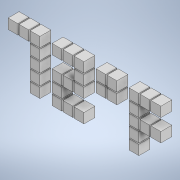
# Autodesk Inventor part: Sun Icon Mockup
Saved by Autodesk Inventor 2020 (Build 240168000, 168)
## iProperties
Created: 2021-04-14
Part Number: Sun Icon Mockup
Material: Generic
Document SubType Name: Modeling
Designer: user
Density: 1 g/cm^3
Appearance: Default
Author: user
Autodesk Inventor part; units mm, degrees
ref_plane "YZ Plane" through (0, 0, 0) normal (1, 0, 0) x (0, 1, 0)
ref_plane "XZ Plane" through (0, 0, 0) normal (0, 1, 0) x (-1, 0, 0)
ref_plane "XY Plane" through (0, 0, 0) normal (0, 0, 1) x (1, 0, 0)
sketch "Sketch1" plane through (0, 0, 0) normal (0, 0, 1) x (1, 0, 0)
  line L0 (0, 0) -> (9, 0)
  line L1 (9, 0) -> (9, 9)
  line L2 (9, 9) -> (0, 9)
  line L3 (0, 9) -> (0, 0)
  line L4 (10, 0) -> (19, 0)
  line L5 (19, 0) -> (19, 9)
  line L6 (10, 9) -> (10, 0)
  line L7 (19, 9) -> (10, 9)
  line L8 (20, 0) -> (29, 0)
  line L9 (29, 0) -> (29, 9)
  line L10 (20, 9) -> (20, 0)
  line L11 (29, 9) -> (20, 9)
  line L12 (30, 0) -> (39, 0)
  line L13 (39, 0) -> (39, 9)
  line L14 (30, 9) -> (30, 0)
  line L15 (39, 9) -> (30, 9)
  line L16 (40, 0) -> (49, 0)
  line L17 (49, 0) -> (49, 9)
  line L18 (40, 9) -> (40, 0)
  line L19 (49, 9) -> (40, 9)
  line L20 (50, 0) -> (59, 0)
  line L21 (59, 0) -> (59, 9)
  line L22 (50, 9) -> (50, 0)
  line L23 (59, 9) -> (50, 9)
  line L24 (60, 0) -> (69, 0)
  line L25 (69, 0) -> (69, 9)
  line L26 (60, 9) -> (60, 0)
  line L27 (69, 9) -> (60, 9)
  line L28 (70, 0) -> (79, 0)
  line L29 (79, 0) -> (79, 9)
  line L30 (70, 9) -> (70, 0)
  line L31 (79, 9) -> (70, 9)
  line L32 (80, 0) -> (89, 0)
  line L33 (89, 0) -> (89, 9)
  line L34 (80, 9) -> (80, 0)
  line L35 (89, 9) -> (80, 9)
  line L36 (90, 0) -> (99, 0)
  line L37 (99, 0) -> (99, 9)
  line L38 (90, 9) -> (90, 0)
  line L39 (99, 9) -> (90, 9)
  line L40 (100, 0) -> (109, 0)
  line L41 (109, 0) -> (109, 9)
  line L42 (100, 9) -> (100, 0)
  line L43 (109, 9) -> (100, 9)
  line L44 (110, 0) -> (119, 0)
  line L45 (119, 0) -> (119, 9)
  line L46 (110, 9) -> (110, 0)
  line L47 (119, 9) -> (110, 9)
  line L48 (120, 0) -> (129, 0)
  line L49 (129, 0) -> (129, 9)
  line L50 (120, 9) -> (120, 0)
  line L51 (129, 9) -> (120, 9)
  line L52 (130, 0) -> (139, 0)
  line L53 (139, 0) -> (139, 9)
  line L54 (130, 9) -> (130, 0)
  line L55 (139, 9) -> (130, 9)
  line L56 (140, 0) -> (149, 0)
  line L57 (149, 0) -> (149, 9)
  line L58 (140, 9) -> (140, 0)
  line L59 (149, 9) -> (140, 9)
  line L60 (150, 0) -> (159, 0)
  line L61 (159, 0) -> (159, 9)
  line L62 (150, 9) -> (150, 0)
  line L63 (159, 9) -> (150, 9)
  line L64 (160, 0) -> (169, 0)
  line L65 (169, 0) -> (169, 9)
  line L66 (160, 9) -> (160, 0)
  line L67 (169, 9) -> (160, 9)
  line L68 (170, 0) -> (179, 0)
  line L69 (179, 0) -> (179, 9)
  line L70 (170, 9) -> (170, 0)
  line L71 (179, 9) -> (170, 9)
  line L72 (180, 0) -> (189, 0)
  line L73 (189, 0) -> (189, 9)
  line L74 (180, 9) -> (180, 0)
  line L75 (189, 9) -> (180, 9)
  line L76 (190, 0) -> (199, 0)
  line L77 (199, 0) -> (199, 9)
  line L78 (190, 9) -> (190, 0)
  line L79 (199, 9) -> (190, 9)
  line L80 (200, 0) -> (209, 0)
  line L81 (209, 0) -> (209, 9)
  line L82 (200, 9) -> (200, 0)
  line L83 (209, 9) -> (200, 9)
  line L84 (210, 0) -> (219, 0)
  line L85 (219, 0) -> (219, 9)
  line L86 (210, 9) -> (210, 0)
  line L87 (219, 9) -> (210, 9)
  line L88 (220, 0) -> (229, 0)
  line L89 (229, 0) -> (229, 9)
  line L90 (220, 9) -> (220, 0)
  line L91 (229, 9) -> (220, 9)
  line L92 (230, 0) -> (239, 0)
  line L93 (239, 0) -> (239, 9)
  line L94 (230, 9) -> (230, 0)
  line L95 (239, 9) -> (230, 9)
  line L96 (240, 0) -> (249, 0)
  line L97 (249, 0) -> (249, 9)
  line L98 (240, 9) -> (240, 0)
  line L99 (249, 9) -> (240, 9)
  line L100 (250, 0) -> (259, 0)
  line L101 (259, 0) -> (259, 9)
  line L102 (250, 9) -> (250, 0)
  line L103 (259, 9) -> (250, 9)
  line L104 (260, 0) -> (269, 0)
  line L105 (269, 0) -> (269, 9)
  line L106 (260, 9) -> (260, 0)
  line L107 (269, 9) -> (260, 9)
  line L108 (270, 0) -> (279, 0)
  line L109 (279, 0) -> (279, 9)
  line L110 (270, 9) -> (270, 0)
  line L111 (279, 9) -> (270, 9)
  line L112 (280, 0) -> (289, 0)
  line L113 (289, 0) -> (289, 9)
  line L114 (280, 9) -> (280, 0)
  line L115 (289, 9) -> (280, 9)
  line L116 (290, 0) -> (299, 0)
  line L117 (299, 0) -> (299, 9)
  line L118 (290, 9) -> (290, 0)
  line L119 (299, 9) -> (290, 9)
  line L120 (300, 0) -> (309, 0)
  line L121 (309, 0) -> (309, 9)
  line L122 (300, 9) -> (300, 0)
  line L123 (309, 9) -> (300, 9)
  line L124 (310, 0) -> (319, 0)
  line L125 (319, 0) -> (319, 9)
  line L126 (310, 9) -> (310, 0)
  line L127 (319, 9) -> (310, 9)
  line L128 (0, -10) -> (9, -10)
  line L129 (9, -10) -> (9, -1)
  line L130 (0, -1) -> (0, -10)
  line L131 (9, -1) -> (0, -1)
  line L132 (10, -10) -> (19, -10)
  line L133 (19, -10) -> (19, -1)
  line L134 (10, -1) -> (10, -10)
  line L135 (19, -1) -> (10, -1)
  line L136 (20, -10) -> (29, -10)
  line L137 (29, -10) -> (29, -1)
  line L138 (20, -1) -> (20, -10)
  line L139 (29, -1) -> (20, -1)
  line L140 (30, -10) -> (39, -10)
  line L141 (39, -10) -> (39, -1)
  line L142 (30, -1) -> (30, -10)
  line L143 (39, -1) -> (30, -1)
  line L144 (40, -10) -> (49, -10)
  line L145 (49, -10) -> (49, -1)
  line L146 (40, -1) -> (40, -10)
  line L147 (49, -1) -> (40, -1)
  line L148 (50, -10) -> (59, -10)
  line L149 (59, -10) -> (59, -1)
  line L150 (50, -1) -> (50, -10)
  line L151 (59, -1) -> (50, -1)
  line L152 (60, -10) -> (69, -10)
  line L153 (69, -10) -> (69, -1)
  line L154 (60, -1) -> (60, -10)
  line L155 (69, -1) -> (60, -1)
  line L156 (70, -10) -> (79, -10)
  line L157 (79, -10) -> (79, -1)
  line L158 (70, -1) -> (70, -10)
  line L159 (79, -1) -> (70, -1)
  line L160 (80, -10) -> (89, -10)
  line L161 (89, -10) -> (89, -1)
  line L162 (80, -1) -> (80, -10)
  line L163 (89, -1) -> (80, -1)
  line L164 (90, -10) -> (99, -10)
  line L165 (99, -10) -> (99, -1)
  line L166 (90, -1) -> (90, -10)
  line L167 (99, -1) -> (90, -1)
  line L168 (100, -10) -> (109, -10)
  line L169 (109, -10) -> (109, -1)
  line L170 (100, -1) -> (100, -10)
  line L171 (109, -1) -> (100, -1)
  line L172 (110, -10) -> (119, -10)
  line L173 (119, -10) -> (119, -1)
  line L174 (110, -1) -> (110, -10)
  line L175 (119, -1) -> (110, -1)
  line L176 (120, -10) -> (129, -10)
  line L177 (129, -10) -> (129, -1)
  line L178 (120, -1) -> (120, -10)
  line L179 (129, -1) -> (120, -1)
  line L180 (130, -10) -> (139, -10)
  line L181 (139, -10) -> (139, -1)
  line L182 (130, -1) -> (130, -10)
  line L183 (139, -1) -> (130, -1)
  line L184 (140, -10) -> (149, -10)
  line L185 (149, -10) -> (149, -1)
  line L186 (140, -1) -> (140, -10)
  line L187 (149, -1) -> (140, -1)
  line L188 (150, -10) -> (159, -10)
  line L189 (159, -10) -> (159, -1)
  line L190 (150, -1) -> (150, -10)
  line L191 (159, -1) -> (150, -1)
  line L192 (160, -10) -> (169, -10)
  line L193 (169, -10) -> (169, -1)
  line L194 (160, -1) -> (160, -10)
  line L195 (169, -1) -> (160, -1)
  line L196 (170, -10) -> (179, -10)
  line L197 (179, -10) -> (179, -1)
  line L198 (170, -1) -> (170, -10)
  line L199 (179, -1) -> (170, -1)
  line L200 (180, -10) -> (189, -10)
  line L201 (189, -10) -> (189, -1)
  line L202 (180, -1) -> (180, -10)
  line L203 (189, -1) -> (180, -1)
  line L204 (190, -10) -> (199, -10)
  line L205 (199, -10) -> (199, -1)
  line L206 (190, -1) -> (190, -10)
  line L207 (199, -1) -> (190, -1)
  line L208 (200, -10) -> (209, -10)
  line L209 (209, -10) -> (209, -1)
  line L210 (200, -1) -> (200, -10)
  line L211 (209, -1) -> (200, -1)
  line L212 (210, -10) -> (219, -10)
  line L213 (219, -10) -> (219, -1)
  line L214 (210, -1) -> (210, -10)
  line L215 (219, -1) -> (210, -1)
  line L216 (220, -10) -> (229, -10)
  line L217 (229, -10) -> (229, -1)
  line L218 (220, -1) -> (220, -10)
  line L219 (229, -1) -> (220, -1)
  line L220 (230, -10) -> (239, -10)
  line L221 (239, -10) -> (239, -1)
  line L222 (230, -1) -> (230, -10)
  line L223 (239, -1) -> (230, -1)
  line L224 (240, -10) -> (249, -10)
  line L225 (249, -10) -> (249, -1)
  line L226 (240, -1) -> (240, -10)
  line L227 (249, -1) -> (240, -1)
  line L228 (250, -10) -> (259, -10)
  line L229 (259, -10) -> (259, -1)
  line L230 (250, -1) -> (250, -10)
  line L231 (259, -1) -> (250, -1)
  line L232 (260, -10) -> (269, -10)
  line L233 (269, -10) -> (269, -1)
  line L234 (260, -1) -> (260, -10)
  line L235 (269, -1) -> (260, -1)
  line L236 (270, -10) -> (279, -10)
  line L237 (279, -10) -> (279, -1)
  line L238 (270, -1) -> (270, -10)
  line L239 (279, -1) -> (270, -1)
  line L240 (280, -10) -> (289, -10)
  line L241 (289, -10) -> (289, -1)
  line L242 (280, -1) -> (280, -10)
  line L243 (289, -1) -> (280, -1)
  line L244 (290, -10) -> (299, -10)
  line L245 (299, -10) -> (299, -1)
  line L246 (290, -1) -> (290, -10)
  line L247 (299, -1) -> (290, -1)
  line L248 (300, -10) -> (309, -10)
  line L249 (309, -10) -> (309, -1)
  line L250 (300, -1) -> (300, -10)
  line L251 (309, -1) -> (300, -1)
  line L252 (310, -10) -> (319, -10)
  line L253 (319, -10) -> (319, -1)
  line L254 (310, -1) -> (310, -10)
  line L255 (319, -1) -> (310, -1)
  line L256 (0, -20) -> (9, -20)
  line L257 (9, -20) -> (9, -11)
  line L258 (0, -11) -> (0, -20)
  line L259 (9, -11) -> (0, -11)
  line L260 (10, -20) -> (19, -20)
  line L261 (19, -20) -> (19, -11)
  line L262 (10, -11) -> (10, -20)
  line L263 (19, -11) -> (10, -11)
  line L264 (20, -20) -> (29, -20)
  line L265 (29, -20) -> (29, -11)
  line L266 (20, -11) -> (20, -20)
  line L267 (29, -11) -> (20, -11)
  line L268 (30, -20) -> (39, -20)
  line L269 (39, -20) -> (39, -11)
  line L270 (30, -11) -> (30, -20)
  line L271 (39, -11) -> (30, -11)
  line L272 (40, -20) -> (49, -20)
  line L273 (49, -20) -> (49, -11)
  line L274 (40, -11) -> (40, -20)
  line L275 (49, -11) -> (40, -11)
  line L276 (50, -20) -> (59, -20)
  line L277 (59, -20) -> (59, -11)
  line L278 (50, -11) -> (50, -20)
  line L279 (59, -11) -> (50, -11)
  line L280 (60, -20) -> (69, -20)
  line L281 (69, -20) -> (69, -11)
  line L282 (60, -11) -> (60, -20)
  line L283 (69, -11) -> (60, -11)
  line L284 (70, -20) -> (79, -20)
  line L285 (79, -20) -> (79, -11)
  line L286 (70, -11) -> (70, -20)
  line L287 (79, -11) -> (70, -11)
  line L288 (80, -20) -> (89, -20)
  line L289 (89, -20) -> (89, -11)
  line L290 (80, -11) -> (80, -20)
  line L291 (89, -11) -> (80, -11)
  line L292 (90, -20) -> (99, -20)
  line L293 (99, -20) -> (99, -11)
  line L294 (90, -11) -> (90, -20)
  line L295 (99, -11) -> (90, -11)
  line L296 (100, -20) -> (109, -20)
  line L297 (109, -20) -> (109, -11)
  line L298 (100, -11) -> (100, -20)
  line L299 (109, -11) -> (100, -11)
  line L300 (110, -20) -> (119, -20)
  line L301 (119, -20) -> (119, -11)
  line L302 (110, -11) -> (110, -20)
  line L303 (119, -11) -> (110, -11)
  line L304 (120, -20) -> (129, -20)
  line L305 (129, -20) -> (129, -11)
  line L306 (120, -11) -> (120, -20)
  line L307 (129, -11) -> (120, -11)
  line L308 (130, -20) -> (139, -20)
  line L309 (139, -20) -> (139, -11)
  line L310 (130, -11) -> (130, -20)
  line L311 (139, -11) -> (130, -11)
  line L312 (140, -20) -> (149, -20)
  line L313 (149, -20) -> (149, -11)
  line L314 (140, -11) -> (140, -20)
  line L315 (149, -11) -> (140, -11)
  line L316 (150, -20) -> (159, -20)
  line L317 (159, -20) -> (159, -11)
  line L318 (150, -11) -> (150, -20)
  line L319 (159, -11) -> (150, -11)
  line L320 (160, -20) -> (169, -20)
  line L321 (169, -20) -> (169, -11)
  line L322 (160, -11) -> (160, -20)
  line L323 (169, -11) -> (160, -11)
  line L324 (170, -20) -> (179, -20)
  line L325 (179, -20) -> (179, -11)
  line L326 (170, -11) -> (170, -20)
  line L327 (179, -11) -> (170, -11)
  line L328 (180, -20) -> (189, -20)
  line L329 (189, -20) -> (189, -11)
  line L330 (180, -11) -> (180, -20)
  line L331 (189, -11) -> (180, -11)
  line L332 (190, -20) -> (199, -20)
  line L333 (199, -20) -> (199, -11)
  line L334 (190, -11) -> (190, -20)
  line L335 (199, -11) -> (190, -11)
  line L336 (200, -20) -> (209, -20)
  line L337 (209, -20) -> (209, -11)
  line L338 (200, -11) -> (200, -20)
  line L339 (209, -11) -> (200, -11)
  line L340 (210, -20) -> (219, -20)
  line L341 (219, -20) -> (219, -11)
  line L342 (210, -11) -> (210, -20)
  line L343 (219, -11) -> (210, -11)
  line L344 (220, -20) -> (229, -20)
  line L345 (229, -20) -> (229, -11)
  line L346 (220, -11) -> (220, -20)
  line L347 (229, -11) -> (220, -11)
  line L348 (230, -20) -> (239, -20)
  line L349 (239, -20) -> (239, -11)
  line L350 (230, -11) -> (230, -20)
  line L351 (239, -11) -> (230, -11)
  line L352 (240, -20) -> (249, -20)
  line L353 (249, -20) -> (249, -11)
  line L354 (240, -11) -> (240, -20)
  line L355 (249, -11) -> (240, -11)
  line L356 (250, -20) -> (259, -20)
  line L357 (259, -20) -> (259, -11)
  line L358 (250, -11) -> (250, -20)
  line L359 (259, -11) -> (250, -11)
  line L360 (260, -20) -> (269, -20)
  line L361 (269, -20) -> (269, -11)
  line L362 (260, -11) -> (260, -20)
  line L363 (269, -11) -> (260, -11)
  line L364 (270, -20) -> (279, -20)
  line L365 (279, -20) -> (279, -11)
  line L366 (270, -11) -> (270, -20)
  line L367 (279, -11) -> (270, -11)
  line L368 (280, -20) -> (289, -20)
  line L369 (289, -20) -> (289, -11)
  line L370 (280, -11) -> (280, -20)
  line L371 (289, -11) -> (280, -11)
  line L372 (290, -20) -> (299, -20)
  line L373 (299, -20) -> (299, -11)
  line L374 (290, -11) -> (290, -20)
  line L375 (299, -11) -> (290, -11)
  line L376 (300, -20) -> (309, -20)
  line L377 (309, -20) -> (309, -11)
  line L378 (300, -11) -> (300, -20)
  line L379 (309, -11) -> (300, -11)
  line L380 (310, -20) -> (319, -20)
  line L381 (319, -20) -> (319, -11)
  line L382 (310, -11) -> (310, -20)
  line L383 (319, -11) -> (310, -11)
  line L384 (0, -30) -> (9, -30)
  line L385 (9, -30) -> (9, -21)
  line L386 (0, -21) -> (0, -30)
  line L387 (9, -21) -> (0, -21)
  line L388 (10, -30) -> (19, -30)
  line L389 (19, -30) -> (19, -21)
  line L390 (10, -21) -> (10, -30)
  line L391 (19, -21) -> (10, -21)
  line L392 (20, -30) -> (29, -30)
  line L393 (29, -30) -> (29, -21)
  line L394 (20, -21) -> (20, -30)
  line L395 (29, -21) -> (20, -21)
  line L396 (30, -30) -> (39, -30)
  line L397 (39, -30) -> (39, -21)
  line L398 (30, -21) -> (30, -30)
  line L399 (39, -21) -> (30, -21)
  line L400 (40, -30) -> (49, -30)
  line L401 (49, -30) -> (49, -21)
  line L402 (40, -21) -> (40, -30)
  line L403 (49, -21) -> (40, -21)
  line L404 (50, -30) -> (59, -30)
  line L405 (59, -30) -> (59, -21)
  line L406 (50, -21) -> (50, -30)
  line L407 (59, -21) -> (50, -21)
  line L408 (60, -30) -> (69, -30)
  line L409 (69, -30) -> (69, -21)
  line L410 (60, -21) -> (60, -30)
  line L411 (69, -21) -> (60, -21)
  line L412 (70, -30) -> (79, -30)
  line L413 (79, -30) -> (79, -21)
  line L414 (70, -21) -> (70, -30)
  line L415 (79, -21) -> (70, -21)
  line L416 (80, -30) -> (89, -30)
  line L417 (89, -30) -> (89, -21)
  line L418 (80, -21) -> (80, -30)
  line L419 (89, -21) -> (80, -21)
  line L420 (90, -30) -> (99, -30)
  line L421 (99, -30) -> (99, -21)
  line L422 (90, -21) -> (90, -30)
  line L423 (99, -21) -> (90, -21)
  line L424 (100, -30) -> (109, -30)
  line L425 (109, -30) -> (109, -21)
  line L426 (100, -21) -> (100, -30)
  line L427 (109, -21) -> (100, -21)
  line L428 (110, -30) -> (119, -30)
  line L429 (119, -30) -> (119, -21)
  line L430 (110, -21) -> (110, -30)
  line L431 (119, -21) -> (110, -21)
  line L432 (120, -30) -> (129, -30)
  line L433 (129, -30) -> (129, -21)
  line L434 (120, -21) -> (120, -30)
  line L435 (129, -21) -> (120, -21)
  line L436 (130, -30) -> (139, -30)
  line L437 (139, -30) -> (139, -21)
  line L438 (130, -21) -> (130, -30)
  line L439 (139, -21) -> (130, -21)
  line L440 (140, -30) -> (149, -30)
  line L441 (149, -30) -> (149, -21)
  line L442 (140, -21) -> (140, -30)
  line L443 (149, -21) -> (140, -21)
  line L444 (150, -30) -> (159, -30)
  line L445 (159, -30) -> (159, -21)
  line L446 (150, -21) -> (150, -30)
  line L447 (159, -21) -> (150, -21)
  line L448 (160, -30) -> (169, -30)
  line L449 (169, -30) -> (169, -21)
  line L450 (160, -21) -> (160, -30)
  line L451 (169, -21) -> (160, -21)
  line L452 (170, -30) -> (179, -30)
  line L453 (179, -30) -> (179, -21)
  line L454 (170, -21) -> (170, -30)
  line L455 (179, -21) -> (170, -21)
  line L456 (180, -30) -> (189, -30)
  line L457 (189, -30) -> (189, -21)
  line L458 (180, -21) -> (180, -30)
  line L459 (189, -21) -> (180, -21)
  line L460 (190, -30) -> (199, -30)
  line L461 (199, -30) -> (199, -21)
  line L462 (190, -21) -> (190, -30)
  line L463 (199, -21) -> (190, -21)
  line L464 (200, -30) -> (209, -30)
  line L465 (209, -30) -> (209, -21)
  line L466 (200, -21) -> (200, -30)
  line L467 (209, -21) -> (200, -21)
  line L468 (210, -30) -> (219, -30)
  line L469 (219, -30) -> (219, -21)
  line L470 (210, -21) -> (210, -30)
  line L471 (219, -21) -> (210, -21)
  line L472 (220, -30) -> (229, -30)
  line L473 (229, -30) -> (229, -21)
  line L474 (220, -21) -> (220, -30)
  line L475 (229, -21) -> (220, -21)
  line L476 (230, -30) -> (239, -30)
  line L477 (239, -30) -> (239, -21)
  line L478 (230, -21) -> (230, -30)
  line L479 (239, -21) -> (230, -21)
  line L480 (240, -30) -> (249, -30)
  line L481 (249, -30) -> (249, -21)
  line L482 (240, -21) -> (240, -30)
  line L483 (249, -21) -> (240, -21)
  line L484 (250, -30) -> (259, -30)
  line L485 (259, -30) -> (259, -21)
  line L486 (250, -21) -> (250, -30)
  line L487 (259, -21) -> (250, -21)
  line L488 (260, -30) -> (269, -30)
  line L489 (269, -30) -> (269, -21)
  line L490 (260, -21) -> (260, -30)
  line L491 (269, -21) -> (260, -21)
  line L492 (270, -30) -> (279, -30)
  line L493 (279, -30) -> (279, -21)
  line L494 (270, -21) -> (270, -30)
  line L495 (279, -21) -> (270, -21)
  line L496 (280, -30) -> (289, -30)
  line L497 (289, -30) -> (289, -21)
  line L498 (280, -21) -> (280, -30)
  line L499 (289, -21) -> (280, -21)
  line L500 (290, -30) -> (299, -30)
  line L501 (299, -30) -> (299, -21)
  line L502 (290, -21) -> (290, -30)
  line L503 (299, -21) -> (290, -21)
  line L504 (300, -30) -> (309, -30)
  line L505 (309, -30) -> (309, -21)
  line L506 (300, -21) -> (300, -30)
  line L507 (309, -21) -> (300, -21)
  line L508 (310, -30) -> (319, -30)
  line L509 (319, -30) -> (319, -21)
  line L510 (310, -21) -> (310, -30)
  line L511 (319, -21) -> (310, -21)
  line L512 (0, -40) -> (9, -40)
  line L513 (9, -40) -> (9, -31)
  line L514 (0, -31) -> (0, -40)
  line L515 (9, -31) -> (0, -31)
  line L516 (10, -40) -> (19, -40)
  line L517 (19, -40) -> (19, -31)
  line L518 (10, -31) -> (10, -40)
  line L519 (19, -31) -> (10, -31)
  line L520 (20, -40) -> (29, -40)
  line L521 (29, -40) -> (29, -31)
  line L522 (20, -31) -> (20, -40)
  line L523 (29, -31) -> (20, -31)
  line L524 (30, -40) -> (39, -40)
  line L525 (39, -40) -> (39, -31)
  line L526 (30, -31) -> (30, -40)
  line L527 (39, -31) -> (30, -31)
  line L528 (40, -40) -> (49, -40)
  line L529 (49, -40) -> (49, -31)
  line L530 (40, -31) -> (40, -40)
  line L531 (49, -31) -> (40, -31)
  line L532 (50, -40) -> (59, -40)
  line L533 (59, -40) -> (59, -31)
  line L534 (50, -31) -> (50, -40)
  line L535 (59, -31) -> (50, -31)
  line L536 (60, -40) -> (69, -40)
  line L537 (69, -40) -> (69, -31)
  line L538 (60, -31) -> (60, -40)
  line L539 (69, -31) -> (60, -31)
  line L540 (70, -40) -> (79, -40)
  line L541 (79, -40) -> (79, -31)
  line L542 (70, -31) -> (70, -40)
  line L543 (79, -31) -> (70, -31)
  line L544 (80, -40) -> (89, -40)
  line L545 (89, -40) -> (89, -31)
  line L546 (80, -31) -> (80, -40)
  line L547 (89, -31) -> (80, -31)
  line L548 (90, -40) -> (99, -40)
  line L549 (99, -40) -> (99, -31)
  line L550 (90, -31) -> (90, -40)
  line L551 (99, -31) -> (90, -31)
  line L552 (100, -40) -> (109, -40)
  line L553 (109, -40) -> (109, -31)
  line L554 (100, -31) -> (100, -40)
  line L555 (109, -31) -> (100, -31)
  line L556 (110, -40) -> (119, -40)
  line L557 (119, -40) -> (119, -31)
  line L558 (110, -31) -> (110, -40)
  line L559 (119, -31) -> (110, -31)
  line L560 (120, -40) -> (129, -40)
  line L561 (129, -40) -> (129, -31)
  line L562 (120, -31) -> (120, -40)
  line L563 (129, -31) -> (120, -31)
  line L564 (130, -40) -> (139, -40)
  line L565 (139, -40) -> (139, -31)
  line L566 (130, -31) -> (130, -40)
  line L567 (139, -31) -> (130, -31)
  line L568 (140, -40) -> (149, -40)
  line L569 (149, -40) -> (149, -31)
  line L570 (140, -31) -> (140, -40)
  line L571 (149, -31) -> (140, -31)
  line L572 (150, -40) -> (159, -40)
  line L573 (159, -40) -> (159, -31)
  line L574 (150, -31) -> (150, -40)
  line L575 (159, -31) -> (150, -31)
  line L576 (160, -40) -> (169, -40)
  line L577 (169, -40) -> (169, -31)
  line L578 (160, -31) -> (160, -40)
  line L579 (169, -31) -> (160, -31)
  line L580 (170, -40) -> (179, -40)
  line L581 (179, -40) -> (179, -31)
  line L582 (170, -31) -> (170, -40)
  line L583 (179, -31) -> (170, -31)
  line L584 (180, -40) -> (189, -40)
  line L585 (189, -40) -> (189, -31)
  line L586 (180, -31) -> (180, -40)
  line L587 (189, -31) -> (180, -31)
  line L588 (190, -40) -> (199, -40)
  line L589 (199, -40) -> (199, -31)
  line L590 (190, -31) -> (190, -40)
  line L591 (199, -31) -> (190, -31)
  line L592 (200, -40) -> (209, -40)
  line L593 (209, -40) -> (209, -31)
  line L594 (200, -31) -> (200, -40)
  line L595 (209, -31) -> (200, -31)
  line L596 (210, -40) -> (219, -40)
  line L597 (219, -40) -> (219, -31)
  line L598 (210, -31) -> (210, -40)
  line L599 (219, -31) -> (210, -31)
  line L600 (220, -40) -> (229, -40)
  line L601 (229, -40) -> (229, -31)
  line L602 (220, -31) -> (220, -40)
  line L603 (229, -31) -> (220, -31)
  line L604 (230, -40) -> (239, -40)
  line L605 (239, -40) -> (239, -31)
  line L606 (230, -31) -> (230, -40)
  line L607 (239, -31) -> (230, -31)
  line L608 (240, -40) -> (249, -40)
  line L609 (249, -40) -> (249, -31)
  line L610 (240, -31) -> (240, -40)
  line L611 (249, -31) -> (240, -31)
  line L612 (250, -40) -> (259, -40)
  line L613 (259, -40) -> (259, -31)
  line L614 (250, -31) -> (250, -40)
  line L615 (259, -31) -> (250, -31)
  line L616 (260, -40) -> (269, -40)
  line L617 (269, -40) -> (269, -31)
  line L618 (260, -31) -> (260, -40)
  line L619 (269, -31) -> (260, -31)
  line L620 (270, -40) -> (279, -40)
  line L621 (279, -40) -> (279, -31)
  line L622 (270, -31) -> (270, -40)
  line L623 (279, -31) -> (270, -31)
  line L624 (280, -40) -> (289, -40)
  line L625 (289, -40) -> (289, -31)
  line L626 (280, -31) -> (280, -40)
  line L627 (289, -31) -> (280, -31)
  line L628 (290, -40) -> (299, -40)
  line L629 (299, -40) -> (299, -31)
  line L630 (290, -31) -> (290, -40)
  line L631 (299, -31) -> (290, -31)
  line L632 (300, -40) -> (309, -40)
  line L633 (309, -40) -> (309, -31)
  line L634 (300, -31) -> (300, -40)
  line L635 (309, -31) -> (300, -31)
  line L636 (310, -40) -> (319, -40)
  line L637 (319, -40) -> (319, -31)
  line L638 (310, -31) -> (310, -40)
  line L639 (319, -31) -> (310, -31)
  line L640 (0, -50) -> (9, -50)
  line L641 (9, -50) -> (9, -41)
  line L642 (0, -41) -> (0, -50)
  line L643 (9, -41) -> (0, -41)
  line L644 (10, -50) -> (19, -50)
  line L645 (19, -50) -> (19, -41)
  line L646 (10, -41) -> (10, -50)
  line L647 (19, -41) -> (10, -41)
  line L648 (20, -50) -> (29, -50)
  line L649 (29, -50) -> (29, -41)
  line L650 (20, -41) -> (20, -50)
  line L651 (29, -41) -> (20, -41)
  line L652 (30, -50) -> (39, -50)
  line L653 (39, -50) -> (39, -41)
  line L654 (30, -41) -> (30, -50)
  line L655 (39, -41) -> (30, -41)
  line L656 (40, -50) -> (49, -50)
  line L657 (49, -50) -> (49, -41)
  line L658 (40, -41) -> (40, -50)
  line L659 (49, -41) -> (40, -41)
  line L660 (50, -50) -> (59, -50)
  line L661 (59, -50) -> (59, -41)
  line L662 (50, -41) -> (50, -50)
  line L663 (59, -41) -> (50, -41)
  line L664 (60, -50) -> (69, -50)
  line L665 (69, -50) -> (69, -41)
  line L666 (60, -41) -> (60, -50)
  line L667 (69, -41) -> (60, -41)
  line L668 (70, -50) -> (79, -50)
  line L669 (79, -50) -> (79, -41)
  line L670 (70, -41) -> (70, -50)
  line L671 (79, -41) -> (70, -41)
  line L672 (80, -50) -> (89, -50)
  line L673 (89, -50) -> (89, -41)
  line L674 (80, -41) -> (80, -50)
  line L675 (89, -41) -> (80, -41)
  line L676 (90, -50) -> (99, -50)
  line L677 (99, -50) -> (99, -41)
  line L678 (90, -41) -> (90, -50)
  line L679 (99, -41) -> (90, -41)
  line L680 (100, -50) -> (109, -50)
  line L681 (109, -50) -> (109, -41)
  line L682 (100, -41) -> (100, -50)
  line L683 (109, -41) -> (100, -41)
  line L684 (110, -50) -> (119, -50)
  line L685 (119, -50) -> (119, -41)
  line L686 (110, -41) -> (110, -50)
  line L687 (119, -41) -> (110, -41)
  line L688 (120, -50) -> (129, -50)
  line L689 (129, -50) -> (129, -41)
  line L690 (120, -41) -> (120, -50)
  line L691 (129, -41) -> (120, -41)
  line L692 (130, -50) -> (139, -50)
  line L693 (139, -50) -> (139, -41)
  line L694 (130, -41) -> (130, -50)
  line L695 (139, -41) -> (130, -41)
  line L696 (140, -50) -> (149, -50)
  line L697 (149, -50) -> (149, -41)
  line L698 (140, -41) -> (140, -50)
  line L699 (149, -41) -> (140, -41)
  line L700 (150, -50) -> (159, -50)
  line L701 (159, -50) -> (159, -41)
  line L702 (150, -41) -> (150, -50)
  line L703 (159, -41) -> (150, -41)
  line L704 (160, -50) -> (169, -50)
  line L705 (169, -50) -> (169, -41)
  line L706 (160, -41) -> (160, -50)
  line L707 (169, -41) -> (160, -41)
  line L708 (170, -50) -> (179, -50)
  line L709 (179, -50) -> (179, -41)
  line L710 (170, -41) -> (170, -50)
  line L711 (179, -41) -> (170, -41)
  line L712 (180, -50) -> (189, -50)
  line L713 (189, -50) -> (189, -41)
  line L714 (180, -41) -> (180, -50)
  line L715 (189, -41) -> (180, -41)
  line L716 (190, -50) -> (199, -50)
  line L717 (199, -50) -> (199, -41)
  line L718 (190, -41) -> (190, -50)
  line L719 (199, -41) -> (190, -41)
  line L720 (200, -50) -> (209, -50)
  line L721 (209, -50) -> (209, -41)
  line L722 (200, -41) -> (200, -50)
  line L723 (209, -41) -> (200, -41)
  line L724 (210, -50) -> (219, -50)
  line L725 (219, -50) -> (219, -41)
  line L726 (210, -41) -> (210, -50)
  line L727 (219, -41) -> (210, -41)
  line L728 (220, -50) -> (229, -50)
  line L729 (229, -50) -> (229, -41)
  line L730 (220, -41) -> (220, -50)
  line L731 (229, -41) -> (220, -41)
  line L732 (230, -50) -> (239, -50)
  line L733 (239, -50) -> (239, -41)
  line L734 (230, -41) -> (230, -50)
  line L735 (239, -41) -> (230, -41)
  line L736 (240, -50) -> (249, -50)
  line L737 (249, -50) -> (249, -41)
  line L738 (240, -41) -> (240, -50)
  line L739 (249, -41) -> (240, -41)
  line L740 (250, -50) -> (259, -50)
  line L741 (259, -50) -> (259, -41)
  line L742 (250, -41) -> (250, -50)
  line L743 (259, -41) -> (250, -41)
  line L744 (260, -50) -> (269, -50)
  line L745 (269, -50) -> (269, -41)
  line L746 (260, -41) -> (260, -50)
  line L747 (269, -41) -> (260, -41)
  line L748 (270, -50) -> (279, -50)
  line L749 (279, -50) -> (279, -41)
  line L750 (270, -41) -> (270, -50)
  line L751 (279, -41) -> (270, -41)
  line L752 (280, -50) -> (289, -50)
  line L753 (289, -50) -> (289, -41)
  line L754 (280, -41) -> (280, -50)
  line L755 (289, -41) -> (280, -41)
  line L756 (290, -50) -> (299, -50)
  line L757 (299, -50) -> (299, -41)
  line L758 (290, -41) -> (290, -50)
  line L759 (299, -41) -> (290, -41)
  line L760 (300, -50) -> (309, -50)
  line L761 (309, -50) -> (309, -41)
  line L762 (300, -41) -> (300, -50)
  line L763 (309, -41) -> (300, -41)
  line L764 (310, -50) -> (319, -50)
  line L765 (319, -50) -> (319, -41)
  line L766 (310, -41) -> (310, -50)
  line L767 (319, -41) -> (310, -41)
  line L768 (0, -60) -> (9, -60)
  line L769 (9, -60) -> (9, -51)
  line L770 (0, -51) -> (0, -60)
  line L771 (9, -51) -> (0, -51)
  line L772 (10, -60) -> (19, -60)
  line L773 (19, -60) -> (19, -51)
  line L774 (10, -51) -> (10, -60)
  line L775 (19, -51) -> (10, -51)
  line L776 (20, -60) -> (29, -60)
  line L777 (29, -60) -> (29, -51)
  line L778 (20, -51) -> (20, -60)
  line L779 (29, -51) -> (20, -51)
  line L780 (30, -60) -> (39, -60)
  line L781 (39, -60) -> (39, -51)
  line L782 (30, -51) -> (30, -60)
  line L783 (39, -51) -> (30, -51)
  line L784 (40, -60) -> (49, -60)
  line L785 (49, -60) -> (49, -51)
  line L786 (40, -51) -> (40, -60)
  line L787 (49, -51) -> (40, -51)
  line L788 (50, -60) -> (59, -60)
  line L789 (59, -60) -> (59, -51)
  line L790 (50, -51) -> (50, -60)
  line L791 (59, -51) -> (50, -51)
  line L792 (60, -60) -> (69, -60)
  line L793 (69, -60) -> (69, -51)
  line L794 (60, -51) -> (60, -60)
  line L795 (69, -51) -> (60, -51)
  line L796 (70, -60) -> (79, -60)
  line L797 (79, -60) -> (79, -51)
  line L798 (70, -51) -> (70, -60)
  line L799 (79, -51) -> (70, -51)
  line L800 (80, -60) -> (89, -60)
  line L801 (89, -60) -> (89, -51)
  line L802 (80, -51) -> (80, -60)
  line L803 (89, -51) -> (80, -51)
  line L804 (90, -60) -> (99, -60)
  line L805 (99, -60) -> (99, -51)
  line L806 (90, -51) -> (90, -60)
  line L807 (99, -51) -> (90, -51)
  line L808 (100, -60) -> (109, -60)
  line L809 (109, -60) -> (109, -51)
  line L810 (100, -51) -> (100, -60)
  line L811 (109, -51) -> (100, -51)
  line L812 (110, -60) -> (119, -60)
  line L813 (119, -60) -> (119, -51)
  line L814 (110, -51) -> (110, -60)
  line L815 (119, -51) -> (110, -51)
  line L816 (120, -60) -> (129, -60)
  line L817 (129, -60) -> (129, -51)
  line L818 (120, -51) -> (120, -60)
  line L819 (129, -51) -> (120, -51)
  line L820 (130, -60) -> (139, -60)
  line L821 (139, -60) -> (139, -51)
  line L822 (130, -51) -> (130, -60)
  line L823 (139, -51) -> (130, -51)
  line L824 (140, -60) -> (149, -60)
  line L825 (149, -60) -> (149, -51)
  line L826 (140, -51) -> (140, -60)
  line L827 (149, -51) -> (140, -51)
  line L828 (150, -60) -> (159, -60)
  line L829 (159, -60) -> (159, -51)
  line L830 (150, -51) -> (150, -60)
  line L831 (159, -51) -> (150, -51)
  line L832 (160, -60) -> (169, -60)
  line L833 (169, -60) -> (169, -51)
  line L834 (160, -51) -> (160, -60)
  line L835 (169, -51) -> (160, -51)
  line L836 (170, -60) -> (179, -60)
  line L837 (179, -60) -> (179, -51)
  line L838 (170, -51) -> (170, -60)
  line L839 (179, -51) -> (170, -51)
  line L840 (180, -60) -> (189, -60)
  line L841 (189, -60) -> (189, -51)
  line L842 (180, -51) -> (180, -60)
  line L843 (189, -51) -> (180, -51)
  line L844 (190, -60) -> (199, -60)
  line L845 (199, -60) -> (199, -51)
  line L846 (190, -51) -> (190, -60)
  line L847 (199, -51) -> (190, -51)
  line L848 (200, -60) -> (209, -60)
  line L849 (209, -60) -> (209, -51)
  line L850 (200, -51) -> (200, -60)
  line L851 (209, -51) -> (200, -51)
  line L852 (210, -60) -> (219, -60)
  line L853 (219, -60) -> (219, -51)
  line L854 (210, -51) -> (210, -60)
  line L855 (219, -51) -> (210, -51)
  line L856 (220, -60) -> (229, -60)
  line L857 (229, -60) -> (229, -51)
  line L858 (220, -51) -> (220, -60)
  line L859 (229, -51) -> (220, -51)
  line L860 (230, -60) -> (239, -60)
  line L861 (239, -60) -> (239, -51)
  line L862 (230, -51) -> (230, -60)
  line L863 (239, -51) -> (230, -51)
  line L864 (240, -60) -> (249, -60)
  line L865 (249, -60) -> (249, -51)
  line L866 (240, -51) -> (240, -60)
  line L867 (249, -51) -> (240, -51)
  line L868 (250, -60) -> (259, -60)
  line L869 (259, -60) -> (259, -51)
  line L870 (250, -51) -> (250, -60)
  line L871 (259, -51) -> (250, -51)
  line L872 (260, -60) -> (269, -60)
  line L873 (269, -60) -> (269, -51)
  line L874 (260, -51) -> (260, -60)
  line L875 (269, -51) -> (260, -51)
  line L876 (270, -60) -> (279, -60)
  line L877 (279, -60) -> (279, -51)
  line L878 (270, -51) -> (270, -60)
  line L879 (279, -51) -> (270, -51)
  line L880 (280, -60) -> (289, -60)
  line L881 (289, -60) -> (289, -51)
  line L882 (280, -51) -> (280, -60)
  line L883 (289, -51) -> (280, -51)
  line L884 (290, -60) -> (299, -60)
  line L885 (299, -60) -> (299, -51)
  line L886 (290, -51) -> (290, -60)
  line L887 (299, -51) -> (290, -51)
  line L888 (300, -60) -> (309, -60)
  line L889 (309, -60) -> (309, -51)
  line L890 (300, -51) -> (300, -60)
  line L891 (309, -51) -> (300, -51)
  line L892 (310, -60) -> (319, -60)
  line L893 (319, -60) -> (319, -51)
  line L894 (310, -51) -> (310, -60)
  line L895 (319, -51) -> (310, -51)
  line L896 (0, -70) -> (9, -70)
  line L897 (9, -70) -> (9, -61)
  line L898 (0, -61) -> (0, -70)
  line L899 (9, -61) -> (0, -61)
  line L900 (10, -70) -> (19, -70)
  line L901 (19, -70) -> (19, -61)
  line L902 (10, -61) -> (10, -70)
  line L903 (19, -61) -> (10, -61)
  line L904 (20, -70) -> (29, -70)
  line L905 (29, -70) -> (29, -61)
  line L906 (20, -61) -> (20, -70)
  line L907 (29, -61) -> (20, -61)
  line L908 (30, -70) -> (39, -70)
  line L909 (39, -70) -> (39, -61)
  line L910 (30, -61) -> (30, -70)
  line L911 (39, -61) -> (30, -61)
  line L912 (40, -70) -> (49, -70)
  line L913 (49, -70) -> (49, -61)
  line L914 (40, -61) -> (40, -70)
  line L915 (49, -61) -> (40, -61)
  line L916 (50, -70) -> (59, -70)
  line L917 (59, -70) -> (59, -61)
  line L918 (50, -61) -> (50, -70)
  line L919 (59, -61) -> (50, -61)
  line L920 (60, -70) -> (69, -70)
  line L921 (69, -70) -> (69, -61)
  line L922 (60, -61) -> (60, -70)
  line L923 (69, -61) -> (60, -61)
  line L924 (70, -70) -> (79, -70)
  line L925 (79, -70) -> (79, -61)
  line L926 (70, -61) -> (70, -70)
  line L927 (79, -61) -> (70, -61)
  line L928 (80, -70) -> (89, -70)
  line L929 (89, -70) -> (89, -61)
  line L930 (80, -61) -> (80, -70)
  line L931 (89, -61) -> (80, -61)
  line L932 (90, -70) -> (99, -70)
  line L933 (99, -70) -> (99, -61)
  line L934 (90, -61) -> (90, -70)
  line L935 (99, -61) -> (90, -61)
  line L936 (100, -70) -> (109, -70)
  line L937 (109, -70) -> (109, -61)
  line L938 (100, -61) -> (100, -70)
  line L939 (109, -61) -> (100, -61)
  line L940 (110, -70) -> (119, -70)
  line L941 (119, -70) -> (119, -61)
  line L942 (110, -61) -> (110, -70)
  line L943 (119, -61) -> (110, -61)
  line L944 (120, -70) -> (129, -70)
  line L945 (129, -70) -> (129, -61)
  line L946 (120, -61) -> (120, -70)
  line L947 (129, -61) -> (120, -61)
  line L948 (130, -70) -> (139, -70)
  line L949 (139, -70) -> (139, -61)
  line L950 (130, -61) -> (130, -70)
  line L951 (139, -61) -> (130, -61)
  line L952 (140, -70) -> (149, -70)
  line L953 (149, -70) -> (149, -61)
  line L954 (140, -61) -> (140, -70)
  line L955 (149, -61) -> (140, -61)
  line L956 (150, -70) -> (159, -70)
  line L957 (159, -70) -> (159, -61)
  line L958 (150, -61) -> (150, -70)
  line L959 (159, -61) -> (150, -61)
  line L960 (160, -70) -> (169, -70)
  line L961 (169, -70) -> (169, -61)
  line L962 (160, -61) -> (160, -70)
  line L963 (169, -61) -> (160, -61)
  line L964 (170, -70) -> (179, -70)
  line L965 (179, -70) -> (179, -61)
  line L966 (170, -61) -> (170, -70)
  line L967 (179, -61) -> (170, -61)
  line L968 (180, -70) -> (189, -70)
  line L969 (189, -70) -> (189, -61)
  line L970 (180, -61) -> (180, -70)
  line L971 (189, -61) -> (180, -61)
  line L972 (190, -70) -> (199, -70)
  line L973 (199, -70) -> (199, -61)
  line L974 (190, -61) -> (190, -70)
  line L975 (199, -61) -> (190, -61)
  line L976 (200, -70) -> (209, -70)
  line L977 (209, -70) -> (209, -61)
  line L978 (200, -61) -> (200, -70)
  line L979 (209, -61) -> (200, -61)
  line L980 (210, -70) -> (219, -70)
  line L981 (219, -70) -> (219, -61)
  line L982 (210, -61) -> (210, -70)
  line L983 (219, -61) -> (210, -61)
  line L984 (220, -70) -> (229, -70)
  line L985 (229, -70) -> (229, -61)
  line L986 (220, -61) -> (220, -70)
  line L987 (229, -61) -> (220, -61)
  line L988 (230, -70) -> (239, -70)
  line L989 (239, -70) -> (239, -61)
  line L990 (230, -61) -> (230, -70)
  line L991 (239, -61) -> (230, -61)
  line L992 (240, -70) -> (249, -70)
  line L993 (249, -70) -> (249, -61)
  line L994 (240, -61) -> (240, -70)
  line L995 (249, -61) -> (240, -61)
  line L996 (250, -70) -> (259, -70)
  line L997 (259, -70) -> (259, -61)
  line L998 (250, -61) -> (250, -70)
  line L999 (259, -61) -> (250, -61)
  line L1000 (260, -70) -> (269, -70)
  line L1001 (269, -70) -> (269, -61)
  line L1002 (260, -61) -> (260, -70)
  line L1003 (269, -61) -> (260, -61)
  line L1004 (270, -70) -> (279, -70)
  line L1005 (279, -70) -> (279, -61)
  line L1006 (270, -61) -> (270, -70)
  line L1007 (279, -61) -> (270, -61)
  line L1008 (280, -70) -> (289, -70)
  line L1009 (289, -70) -> (289, -61)
  line L1010 (280, -61) -> (280, -70)
  line L1011 (289, -61) -> (280, -61)
  line L1012 (290, -70) -> (299, -70)
  line L1013 (299, -70) -> (299, -61)
  line L1014 (290, -61) -> (290, -70)
  line L1015 (299, -61) -> (290, -61)
  line L1016 (300, -70) -> (309, -70)
  line L1017 (309, -70) -> (309, -61)
  line L1018 (300, -61) -> (300, -70)
  line L1019 (309, -61) -> (300, -61)
  line L1020 (310, -70) -> (319, -70)
  line L1021 (319, -70) -> (319, -61)
  line L1022 (310, -61) -> (310, -70)
  line L1023 (319, -61) -> (310, -61)
  dimension "d0" = 9
  dimension "d1" = 9
  dimension "d4" = 10
  dimension "d7" = 10
  constraints: 2048 end point, 2 collinear, 2 horizontal, 2 parallel, 1 perpendicular, 1 vertical, 2038 other
  measures "d0" distance of L2.end L1.end
  measures "d1" distance of L1.end L0.end
  measures "d4" distance of L1.end L5.end
  measures "d7" distance of L1.end L129.end
extrude "Extrusion1" add sketch "Sketch1" along normal blind 10 contours L190 L191 L189 L188 | L194 L195 L193 L192 | L198 L199 L197 L196 | L206 L207 L205 L204 | L210 L211 L209 L208 | L214 L215 L213 L212 | L222 L223 L221 L220 | L226 L227 L225 L224 | L234 L235 L233 L232 | L238 L239 L237 L236 | L242 L243 L241 L240 | L326 L327 L325 L324 | L342 L343 L341 L340 | L350 L351 L349 L348 | L354 L355 L353 L352 | L362 L363 L361 L360 | L454 L455 L453 L452 | L462 L463 L461 L460 | L466 L467 L465 L464 | L470 L471 L469 L468 | L490 L491 L489 L488 | L494 L495 L493 L492 | L498 L499 L497 L496 | L582 L583 L581 L580 | L590 L591 L589 L588 | L618 L619 L617 L616 | L710 L711 L709 L708 | L718 L719 L717 L716 | L722 L723 L721 L720 | L726 L727 L725 L724 | L746 L747 L745 L744
body "Solid1"
